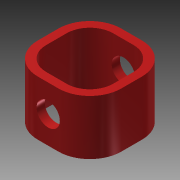
# Autodesk Inventor part: ForkSleeve
Saved by Autodesk Inventor 2014 SP1 (Build 180222100, 222)
## iProperties
Created: 2017-01-18
Part Number: ForkSleeve
Material: Generic
Document SubType Name: Modeling
Designer: danielsikar
Density: 1 g/cm^3
Appearance: Light Red
Author: danielsikar
Autodesk Inventor part; units mm, degrees
ref_plane "YZ Plane" through (0, 0, 0) normal (1, 0, 0) x (0, 1, 0)
ref_plane "XZ Plane" through (0, 0, 0) normal (0, 1, 0) x (-1, 0, 0)
ref_plane "XY Plane" through (0, 0, 0) normal (0, 0, 1) x (1, 0, 0)
ref_plane "Work Plane1" through (-1.5, -4.1, 0) normal (0, -1, 0) x (1, 0, 0)
sketch "Sketch2" plane through (-1.5, -4.1, 0) normal (0, -1, 0) x (1, 0, 0)
  spline S0 degree 3 poles (-0.2, -4) (-0.2, -4.2199) (-0.155, -4.4494) (0.0197, -4.8659) (0.1494, -5.0536) (0.4457, -5.3499) (0.6336, -5.4801) (1.0512, -5.6552) (1.2812, -5.7) (1.7188, -5.7) (1.9488, -5.6552) (2.3664, -5.4801) (2.5543, -5.3499) (2.8506, -5.0536) (2.9803, -4.8659) (3.155, -4.4494) (3.2, -4.2199) (3.2, -3.7801) (3.155, -3.5506) (2.9803, -3.1341) (2.8506, -2.9464) (2.5543, -2.6501) (2.3664, -2.5199) (1.9488, -2.3448) (1.7188, -2.3) (1.2812, -2.3) (1.0512, -2.3448) (0.6336, -2.5199) (0.4457, -2.6501) (0.1494, -2.9464) (0.0197, -3.1341) (-0.155, -3.5506) (-0.2, -3.7801) (-0.2, -4) knots 0 0 0 0 0.065958 0.065958 0.131917 0.131917 0.197553 0.197553 0.263189 0.263189 0.328824 0.328824 0.39446 0.39446 0.460419 0.460419 0.526377 0.526377 0.592335 0.592335 0.658294 0.658294 0.72393 0.72393 0.789566 0.789566 0.855201 0.855201 0.920837 0.920837 0.986796 0.986796 1.052754 1.052754 1.052754 1.052754 projected
  point P0 (1.5, 0)
  point P1 (-0.2, -4)
extrude "Extrusion2" [suppressed]
ref_plane "Work Plane2" through (0, 0, 0) normal (0, 0, 1) x (1, 0, 0)
sketch "Sketch3" plane through (0, 0, 0) normal (0, 0, 1) x (1, 0, 0)
  arc A0 (4.5, 3.5) -> (1.5, 6.5) centre (1.5, 3.5) ccw projected
  line L0 (-1.5, 6.5) -> (1.5, 6.5) projected
  arc A1 (-1.5, 6.5) -> (-4.5, 3.5) centre (-1.5, 3.5) ccw projected
  line L1 (-4.5, 0.5) -> (-4.5, 3.5) projected
  arc A2 (-4.5, 0.5) -> (-1.5, -2.5) centre (-1.5, 0.5) ccw projected
  line L2 (-1.5, -2.5) -> (1.5, -2.5) projected
  arc A3 (1.5, -2.5) -> (4.5, 0.5) centre (1.5, 0.5) ccw projected
  line L3 (4.5, 0.5) -> (4.5, 3.5) projected
  arc A4 (4.9, 3.5) -> (1.5, 6.9) centre (1.5, 3.5) ccw
  line L4 (4.9, 3.5) -> (4.9, 0.5)
  arc A5 (1.5, -2.9) -> (4.9, 0.5) centre (1.5, 0.5) ccw
  line L5 (1.5, -2.9) -> (-1.5, -2.9)
  arc A6 (-4.9, 0.5) -> (-1.5, -2.9) centre (-1.5, 0.5) ccw
  line L6 (-4.9, 0.5) -> (-4.9, 3.5)
  arc A7 (-1.5, 6.9) -> (-4.9, 3.5) centre (-1.5, 3.5) ccw
  line L7 (-1.5, 6.9) -> (1.5, 6.9)
  arc A8 (4.6244, 6.5387) -> (-4.6244, 6.5387) centre (0, 2) ccw projected
  arc A9 (-4.6244, -2.5387) -> (4.6244, -2.5387) centre (0, 2) ccw projected
  line L8 (4.6244, 6.5387) -> (16.8276, 5.0059) projected
  line L9 (-16.8276, 5.0059) -> (-4.6244, 6.5387) projected
  line L10 (-4.6244, -2.5387) -> (-16.8276, -1.0059) projected
  line L11 (16.8276, -1.0059) -> (4.6244, -2.5387) projected
  line L12 (-6.4, 5.9125) -> (-4.4339, 6.1595)
  arc A10 (4.4339, 6.1595) -> (-4.4339, 6.1595) centre (0, 2) ccw
  line L13 (4.4339, 6.1595) -> (6.4, 5.9125)
  line L14 (6.4, -1.9125) -> (4.4339, -2.1595)
  arc A11 (-4.4339, -2.1595) -> (4.4339, -2.1595) centre (0, 2) ccw
  line L15 (-4.4339, -2.1595) -> (-6.4, -1.9125)
  line L16 (-6.4, 5.9125) -> (-6.4, -1.9125)
  line L17 (6.4, 7.8774) -> (6.4, -1.9125)
  point P0 (0, 0)
  dimension "d11" = 0.4
  dimension "d12" = 0.4
  dimension "d13" = 0.4
  dimension "d14" = 1.5
  dimension "d15" = 1.5
  constraints: 20 end point, 12 point on circle, 6 centre point, 1 parallel, 1 perpendicular, 1 point on line, 7 other
  measures "d11" distance between parallel lines of L7 L0
  measures "d12" radial gap between concentric circles of A10 A8
  measures "d13" radial gap between concentric circles of A9 A11
  measures "d14" distance between parallel lines of L6 L16
  measures "d15" distance between parallel lines of L4 L17
extrude "Extrusion3" add sketch "Sketch3" against normal blind 8 contours L12 A10 L13 L17 L14 A11 L15 L16
sketch "Sketch4" plane through (-1.5, -4.1, 0) normal (0, -1, 0) x (1, 0, 0)
  spline S0 degree 3 poles (1.5, -5.7) (1.3275, -5.7) (1.1181, -5.6754) (0.6916, -5.5097) (0.5007, -5.3882) (0.1885, -5.1059) (0.0477, -4.9049) (-0.1308, -4.5285) (-0.1847, -4.2982) (-0.21, -3.8889) (-0.1774, -3.6585) (-0.0472, -3.2645) (0.0654, -3.0658) (0.3443, -2.7324) (0.5358, -2.585) (0.9179, -2.3872) (1.1453, -2.3251) (1.5634, -2.2878) (1.7924, -2.3122) (2.1772, -2.4295) (2.3685, -2.5172) (2.7425, -2.8182) (2.892, -3.0019) (3.1005, -3.3848) (3.1682, -3.611) (3.2151, -4.0563) (3.1829, -4.2987) (3.0681, -4.6965) (2.9478, -4.9082) (2.6974, -5.2274) (2.5158, -5.3795) (2.2209, -5.5443) (2.0954, -5.6019) (1.7867, -5.6811) (1.6425, -5.7) (1.5, -5.7) knots 0 0 0 0 0.051738 0.051738 0.093583 0.093583 0.143159 0.143159 0.198115 0.198115 0.257657 0.257657 0.318526 0.318526 0.385513 0.385513 0.456469 0.456469 0.528586 0.528586 0.590725 0.590725 0.645004 0.645004 0.701391 0.701391 0.762201 0.762201 0.839148 0.839148 0.933962 0.933962 0.986797 0.986797 1.029532 1.029532 1.029532 1.029532 projected
  point P0 (1.5, 0)
  point P1 (1.5, -5.7)
extrude "Extrusion4" cut sketch "Sketch4" against normal through all
body "Solid1"
